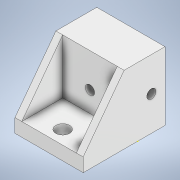
# Autodesk Inventor part: UnionLlantaOmega2
Saved by Autodesk Inventor 2021 (Build 250183000, 183)
## iProperties
Created: 2020-11-13
Part Number: UnionLlantaOmega2
Material: Plástico ABS
Document SubType Name: Modeling
Designer: juanm
Density: 1.06 g/cm^3
Appearance: Suave - Blanco
Author: juanm
Autodesk Inventor part; units mm, degrees
ref_plane "YZ Plane" through (0, 0, 0) normal (1, 0, 0) x (0, 1, 0)
ref_plane "XZ Plane" through (0, 0, 0) normal (0, 1, 0) x (-1, 0, 0)
ref_plane "XY Plane" through (0, 0, 0) normal (0, 0, 1) x (1, 0, 0)
sketch "Boceto1" plane through (0, 0, 0) normal (0, 0, 1) x (1, 0, 0)
  line L0 (0, 0) -> (50, 0)
  line L1 (50, 0) -> (50, 50)
  line L2 (50, 50) -> (0, 50)
  line L3 (0, 50) -> (0, 0)
  line L4 (50, 0) -> (0, 0)
  line L5 (0, 0) -> (0, 10)
  line L6 (0, 10) -> (50, 10)
  line L7 (50, 10) -> (50, 0)
  dimension "d0" = 50
  dimension "d1" = 50
  dimension "d2" = 10
  constraints: 16 end point, 4 parallel, 2 horizontal, 2 perpendicular, 1 point on line
  measures "d0" distance of L2.end L1.end
  measures "d1" distance of L1.end L0.end
  measures "d2" distance of L4.end L5.end
extrude "Extrusión1" add sketch "Boceto1" along normal blind 10
sketch "Boceto2" plane through (0, 0, 10) normal (0, 0, 1) x (1, 0, 0)
  line L0 (0, 0) -> (50, 0) projected
  line L1 (0, 50) -> (0, 0) projected
  line L2 (50, 0) -> (0, 0)
  line L3 (0, 0) -> (0, 10)
  line L4 (0, 10) -> (50, 10)
  line L5 (50, 10) -> (50, 0)
  dimension "d5" = 10
  constraints: 8 end point, 2 parallel, 1 horizontal, 1 perpendicular, 1 point on line
  measures "d5" distance of L2.end L3.end
extrude "Extrusión2" add sketch "Boceto2" along normal blind 30
sketch "Boceto3" plane through (0, 0, 10) normal (0, 0, 1) x (1, 0, 0)
  circle A0 centre (25, 25) radius 3.4
  line L0 (0, 50) -> (0, 10) projected
  line L1 (0, 0) -> (50, 0) projected
  dimension "d8" = 6.8
  dimension "d9" = 25
  dimension "d10" = 25
  constraints: 1 centre point
  measures "d8" diameter of A0
  measures "d9" distance from line of L0 A0.centre
  measures "d10" distance from line of L1 A0.centre
extrude "Extrusión3" cut sketch "Boceto3" against normal blind 10
sketch "Boceto4" plane through (0, 10, 10) normal (0, 1, 0) x (1, 0, 0)
  circle A0 centre (25, -20) radius 5.1
  line L0 (50, 10) -> (0, 10) projected
  line L1 (0, 0) -> (0, -30) projected
  dimension "d13" = 10.2
  dimension "d14" = 30
  dimension "d15" = 25
  constraints: 1 centre point
  measures "d13" diameter of A0
  measures "d14" distance from line of L0 A0.centre
  measures "d15" distance from line of L1 A0.centre
extrude "Extrusión4" cut sketch "Boceto4" against normal blind 10
sketch "Boceto5" plane through (0, 0, 0) normal (-1, 0, 0) x (0, 0, 1)
  line L0 (0, 50) -> (10, 50) projected
  line L1 (10, 10) -> (40, 10) projected
  line L2 (10, 50) -> (40, 10)
  line L3 (40, 10) -> (10, 10)
  line L4 (10, 10) -> (10, 50)
  line L5 (10, 50) -> (10, 10) projected
  point P0 (0, 0)
  constraints: 6 end point, 1 collinear, 1 horizontal, 1 point on line
extrude "Extrusión5" add sketch "Boceto5" against normal blind 5
sketch "Boceto6" plane through (50, 0, 0) normal (1, 0, 0) x (0, 0, -1)
  line L0 (-10, 50) -> (-40, 10) projected
  line L1 (-10, 10) -> (-40, 10) projected
  line L2 (-10, 50) -> (-40, 10)
  line L3 (-40, 10) -> (-10, 10)
  line L4 (-10, 50) -> (-10, 10) projected
  line L5 (-10, 10) -> (-10, 50)
  point P0 (0, 0)
  constraints: 6 end point, 1 collinear, 1 perpendicular
sketch "Boceto7" plane through (50, 0, 0) normal (1, 0, 0) x (0, 0, -1)
  point P0 (0, 0)
sketch "Boceto8" plane through (0, 0, 10) normal (0, 0, 1) x (1, 0, 0)
  point P0 (0, 0)
extrude "Extrusión6" add sketch "Boceto6" against normal blind 5
sketch "Boceto9" plane through (0, 0, 0) normal (0, 0, -1) x (-1, 0, 0)
  line L0 (-5, 5) -> (-45, 5)
  line L1 (-45, 5) -> (-45, 45)
  line L2 (-45, 45) -> (-5, 45)
  line L3 (-5, 45) -> (-5, 5)
  line L4 (-50, 0) -> (-50, 50) projected
  line L5 (-50, 50) -> (0, 50) projected
  line L6 (0, 50) -> (0, 0) projected
  line L7 (0, 0) -> (-50, 0)
  line L8 (-50, 0) -> (-50, 50)
  line L9 (-50, 50) -> (0, 50)
  line L10 (0, 50) -> (0, 0)
  constraints: 16 end point, 4 parallel, 2 horizontal, 2 perpendicular
extrude "Extrusión7" add sketch "Boceto9" along normal blind 20
sketch "Boceto10" plane through (50, 0, 40) normal (1, 0, 0) x (0, 0, -1)
  line L0 (0, 0) -> (0, 10) projected
  circle A0 centre (50, 25) radius 3.375
  line L1 (60, 0) -> (0, 0) projected
  line L2 (60, 50) -> (60, 0) projected
  point P0 (40, 0)
  dimension "d28" = 40
  dimension "d29" = 6.75
  constraints: 1 centre point
  measures "d28" distance from line of L0 point (40, 0)
  measures "d29" diameter of A0
sketch "Boceto12" plane through (0, 0, 40) normal (-1, 0, 0) x (0, 0, 1)
  circle A0 centre (-50, 25) radius 3.375
  line L0 (-60, 0) -> (-60, 50) projected
  line L1 (-30, 50) -> (-60, 50) projected
  point P0 (-40, 0)
  dimension "d35" = 6.75
  constraints: 1 centre point
  measures "d35" diameter of A0
extrude "Extrusión9" cut sketch "Boceto10" against normal blind 5
extrude "Extrusión11" cut sketch "Boceto12" against normal blind 5
